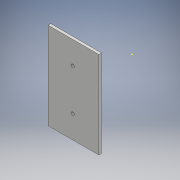
# Autodesk Inventor part: Base
Saved by Autodesk Inventor 2017 (Build 210142000, 142)
## iProperties
Created: 2017-04-26
Part Number: Base
Material: Generic
Document SubType Name: Modeling
Designer: Parshant Bombhi
Density: 1 g/cm^3
Appearance: Default
DistanceOfHolesFromEdge: 2.362 in
Author: Parshant Bombhi
Autodesk Inventor part; units mm, degrees
ref_plane "YZ Plane" through (0, 0, 0) normal (1, 0, 0) x (0, 1, 0)
ref_plane "XZ Plane" through (0, 0, 0) normal (0, 1, 0) x (-1, 0, 0)
ref_plane "XY Plane" through (0, 0, 0) normal (0, 0, 1) x (1, 0, 0)
sketch "Sketch1" plane through (0, 0, 0) normal (0, 1, 0) x (-1, 0, 0)
  line L0 (0, 0) -> (279.4, 0)
  line L1 (212.9145, -36.6988) -> (79.5645, -36.6988)
  line L2 (79.5645, -36.6988) -> (79.5645, -265.2988)
  line L3 (79.5645, -265.2988) -> (212.9145, -265.2988)
  line L4 (212.9145, -265.2988) -> (212.9145, -36.6988)
  dimension "d2" = 228.6
  dimension "d3" = 133.35
  constraints: 10 end point, 2 horizontal, 2 parallel, 1 perpendicular
  measures "d2" distance of L1.end L2.end
  measures "d3" distance of L2.end L3.end
extrude "Extrusion1" add sketch "Sketch1" along normal blind 7
sketch "Sketch2" plane through (0, 7, 0) normal (0, 1, 0) x (1, 0, 0)
  circle A0 centre (-147.9145, 96.6988) radius 3.9688
  circle A1 centre (-147.9145, 205.2988) radius 3.9688
  line L0 (-212.9145, 265.2988) -> (-212.9145, 36.6988) projected
  line L1 (-212.9145, 36.6988) -> (-79.5645, 36.6988) projected
  line L2 (-79.5645, 265.2988) -> (-212.9145, 265.2988) projected
  point P0 (0, 0)
  dimension "d6" = 7.9375
  dimension "d7" = 7.9375
  dimension "d8" = 65
  dimension "d9" = 65
  dimension "DistanceOfHolesFromEdge" = 60
  dimension "d11" = 60
  constraints: 2 centre point
  measures "d6" diameter of A0
  measures "d7" diameter of A1
  measures "d8" distance from line of L0 A0.centre
  measures "d9" distance from line of A1.centre L0
  measures "DistanceOfHolesFromEdge" distance from line of A0.centre L1
  measures "d11" distance from line of A1.centre L2
extrude "Extrusion2" cut sketch "Sketch2" against normal blind 52.75
sketch "Sketch3" plane through (0, 7, 0) normal (0, 1, 0) x (1, 0, 0)
  line L0 (-154.869, 149.729) -> (-139.5444, 149.729) construction
  line L1 (-139.5444, 149.729) -> (-139.5444, 146.1553) construction
  line L2 (-139.5444, 146.1553) -> (-154.869, 146.1553) construction
  line L3 (-154.869, 146.1553) -> (-154.869, 149.729) construction
  point P0 (0, 0)
  constraints: 2 other
equation "\"d7\" = d6"
equation "\"d9\" = d8"
equation "\"d11\" = DistanceOfHolesFromEdge"
body "Solid1"
